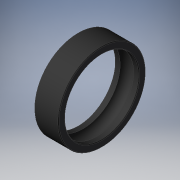
# Autodesk Inventor part: 040102DR-18-H8_or
Saved by Autodesk Inventor 2024 (Build 280153000, 153)
## iProperties
Created: 2023-06-20
Part Number: 040102DR-18-H8_or
Material: Generic
Catalog Web Link: www.cadenas.de
Description: DR-H or-D-Series bearings
Vendor: TOKBEARING
Document SubType Name: Modeling
Designer: psAdmin
Manufacturer: TOKBEARING
Mass: 8700 g
Surface Area: 6.90951 cm^2
Volume: 0.285101 cm^3
Density: 1 g/cm^3
Appearance: PSOLRGB-175-175-175
Category: PARTsolutions
Company: TOKBEARING
PSOL_IDENT_0: {$CADENAS_DATA/23d-libs/tok_bearing/d_series_bearings/dr_h/dr_h_or.prj},177 {VTYP=3D},{NB=040102DR-1
PSOL_IDENT_1: 8-H8_or},{LINA=040102DR-18-H8_or},{NN=DR-H or},{DATE=16.12.2020 00:38:04},{GEOMDATE=19.02.2013 00:00
PSOL_IDENT_2: :00},{VERSION=},{LINEID=1710},{WBVAR=},{WBNUMERIC=}  {NB=040102DR-18-H8_or},{LINA=040102DR-18-H8_or}
PSOL_IDENT_3: ,{KT=DUMMY},{IDNR=},{CODE=040102},{PN=DR-18-H8},{D=18},{SD=8.0},{W=5.0},{W1=-},{W1X=0.000},{W2=-},{W
PSOL_IDENT_4: 2X=0.000},{LOAD=49 (5)},{TYPE=11},{QTY=3.000},{GW=8.7},{BD=3.2},{OP=42.704},{N=6},{R=6.8},{GP=1.4}
NB: 040102DR-18-H8_or
NN: DR-H or
NT: D-Series bearings
NBSYN: $CODE.$PN._or
LINA: 040102DR-18-H8_or
CATALOG: TOK, Inc
CODE: 040102
PN: DR-18-H8
D: 18
SD: 8
W: 5
W1: -
W2: -
LOAD: 49 (5)
TYPE: 11
QTY: 3.000
GW: 8.7
SUPPLIER: TOKBEARING
ARTICLENO: 040102DR-18-H8_or
BOMINFO: 040102DR-18-H8_or
CREATOR: CADENAS GmbH
Title: 040102DR-18-H8_or
Author: Cadenas PARTsolutions
Comments: D-Series bearings
Autodesk Inventor part; units mm, degrees
sketch "Sketch_3" plane through (0, 0, 0) normal (0, 0, 1) x (1, 0, 0)
  line L0 (5, 0) -> (0, 0)
  line L1 (0, 8.875) -> (0, 7.725)
  line L2 (0, 7.725) -> (0.125, 7.6)
  line L3 (0.125, 7.6) -> (1.1144, 7.6)
  arc A0 (3.8856, 7.6) -> (1.1144, 7.6) centre (2.5, 6.8) ccw
  line L4 (3.8856, 7.6) -> (4.875, 7.6)
  line L5 (4.875, 7.6) -> (5, 7.725)
  line L6 (5, 7.725) -> (5, 8.875)
  line L7 (5, 8.875) -> (4.875, 9)
  line L8 (4.875, 9) -> (0.125, 9)
  line L9 (0.125, 9) -> (0, 8.875)
  constraints: 20 end point, 2 point on circle, 1 centre point
revolve "Revolution1" add sketch "Sketch_3" angle 360 about axis through (5, 0, 0) along (1, 0, 0)
ref_plane "OR_Cage_XY" through (0, 0, 0) normal (1, 0, 0) x (0, 0, -1)
ref_plane "OR_Cage_YZ" through (0, 0, 0) normal (0, 0, -1) x (0, 1, 0)
ref_plane "OR_Cage_ZX" through (0, 0, 0) normal (0, 1, 0) x (1, 0, 0)
ref_plane "OR_IR_XY" through (0, 0, 0) normal (1, 0, 0) x (0, 0, -1)
ref_plane "OR_IR_YZ" through (0, 0, 0) normal (0, 0, -1) x (0, 1, 0)
ref_plane "OR_IR_ZX" through (0, 0, 0) normal (0, 1, 0) x (1, 0, 0)
ref_plane "OR_ball_1_XY" through (2.5, 6.8, 0) normal (1, 0, 0) x (0, 0, -1)
ref_plane "OR_ball_1_YZ" through (2.5, 6.8, 0) normal (0, 0, -1) x (0, 1, 0)
ref_plane "OR_ball_1_ZX" through (2.5, 6.8, 0) normal (0, 1, 0) x (1, 0, 0)
ref_plane "OR_ball_2_XY" through (2.5, 3.4, 5.889) normal (1, 0, 0) x (0, 0, -1)
ref_plane "OR_ball_2_YZ" through (2.5, 3.4, 5.889) normal (0, 0, -1) x (0, 1, 0)
ref_plane "OR_ball_2_ZX" through (2.5, 3.4, 5.889) normal (0, 1, 0) x (1, 0, 0)
ref_plane "OR_ball_3_XY" through (2.5, -3.4, 5.889) normal (1, 0, 0) x (0, 0, -1)
ref_plane "OR_ball_3_YZ" through (2.5, -3.4, 5.889) normal (0, 0, -1) x (0, 1, 0)
ref_plane "OR_ball_3_ZX" through (2.5, -3.4, 5.889) normal (0, 1, 0) x (1, 0, 0)
ref_plane "OR_ball_4_XY" through (2.5, -6.8, 0) normal (1, 0, 0) x (0, 0, -1)
ref_plane "OR_ball_4_YZ" through (2.5, -6.8, 0) normal (0, 0, -1) x (0, 1, 0)
ref_plane "OR_ball_4_ZX" through (2.5, -6.8, 0) normal (0, 1, 0) x (1, 0, 0)
ref_plane "OR_ball_5_XY" through (2.5, -3.4, -5.889) normal (1, 0, 0) x (0, 0, -1)
ref_plane "OR_ball_5_YZ" through (2.5, -3.4, -5.889) normal (0, 0, -1) x (0, 1, 0)
ref_plane "OR_ball_5_ZX" through (2.5, -3.4, -5.889) normal (0, 1, 0) x (1, 0, 0)
ref_plane "OR_ball_6_XY" through (2.5, 3.4, -5.889) normal (1, 0, 0) x (0, 0, -1)
ref_plane "OR_ball_6_YZ" through (2.5, 3.4, -5.889) normal (0, 0, -1) x (0, 1, 0)
ref_plane "OR_ball_6_ZX" through (2.5, 3.4, -5.889) normal (0, 1, 0) x (1, 0, 0)
body "Solid1"
